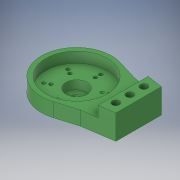
# Autodesk Inventor part: 000.403 - Рычаг
Saved by Autodesk Inventor 2019 (Build 230136000, 136)
## iProperties
Created: 2020-02-28
Part Number: 000.403 - Рычаг
Material: Пластик АБС
Document SubType Name: Modeling
Designer: Петров Иван
Density: 1.06 g/cm^3
Appearance: Гладкий — темный травянисто-зеленый
Author: Петров Иван
Autodesk Inventor part; units mm, degrees
ref_plane "YZ Plane" through (0, 0, 0) normal (1, 0, 0) x (0, 1, 0)
ref_plane "XZ Plane" through (0, 0, 0) normal (0, 1, 0) x (-1, 0, 0)
ref_plane "XY Plane" through (0, 0, 0) normal (0, 0, 1) x (1, 0, 0)
sketch "Эскиз1" plane through (0, 0, 0) normal (0, 1, 0) x (-1, 0, 0)
  arc A0 (13.2517, 5.1196) -> (11.6396, 8.8847) centre (11.8859, 6.7625) ccw
  line L0 (11.6396, 8.8847) -> (3.5765, 5.9707)
  line L1 (3.5765, 5.9707) -> (2.1921, 14.0362)
  arc A1 (2.1921, 14.0362) -> (-1.8746, 14.5225) centre (0.0865, 13.6747) ccw
  line L2 (-1.8746, 14.5225) -> (-3.3825, 6.0827)
  line L3 (-3.3825, 6.0827) -> (-11.0596, 8.9165)
  arc A2 (-11.0596, 8.9165) -> (-13.5142, 5.6378) centre (-11.7994, 6.9122) ccw
  line L4 (-13.5142, 5.6378) -> (-6.959, 0.112)
  line L5 (-6.959, 0.112) -> (-13.2517, -5.1196)
  arc A3 (-13.2517, -5.1196) -> (-11.6396, -8.8847) centre (-11.8859, -6.7625) ccw
  line L6 (-11.6396, -8.8847) -> (-3.5765, -5.9707)
  line L7 (-3.5765, -5.9707) -> (-2.1921, -14.0362)
  arc A4 (-2.1921, -14.0362) -> (1.8746, -14.5225) centre (-0.0865, -13.6747) ccw
  line L8 (1.8746, -14.5225) -> (3.3825, -6.0827)
  line L9 (3.3825, -6.0827) -> (11.0596, -8.9165)
  arc A5 (11.0596, -8.9165) -> (13.5142, -5.6378) centre (11.7994, -6.9122) ccw
  line L10 (13.5142, -5.6378) -> (6.959, -0.112)
  line L11 (6.959, -0.112) -> (13.2517, 5.1196)
  circle A6 centre (6.6709, 3.7954) radius 1
  circle A7 centre (11.8859, 6.7625) radius 1
  circle A8 centre (9.2109, -5.3958) radius 1
  circle A9 centre (-0.0485, -7.6748) radius 1
  circle A10 centre (-0.0865, -13.6747) radius 1
  circle A11 centre (-9.2784, -5.2789) radius 1
  circle A12 centre (-6.6223, 3.8794) radius 1
  circle A13 centre (-11.7994, 6.9122) radius 1
  circle A14 centre (0.0675, 10.6748) radius 1
  circle A15 centre (0, 0) radius 4.75
  circle A16 centre (0.0865, 13.6747) radius 1
  circle A17 centre (0.0485, 7.6748) radius 1
  circle A18 centre (-9.2109, 5.3958) radius 1
  circle A19 centre (-11.8859, -6.7625) radius 1
  circle A20 centre (-6.6709, -3.7954) radius 1
  circle A21 centre (-0.0675, -10.6748) radius 1
  circle A22 centre (11.7994, -6.9122) radius 1
  circle A23 centre (6.6223, -3.8794) radius 1
  circle A24 centre (9.2784, 5.2789) radius 1
  circle A25 centre (0, 0) radius 1.875
  circle A26 centre (0, 0) radius 20
  circle A27 centre (0, 0) radius 17.5
  point P0 (0, 0)
  dimension "d0" = 40
  dimension "d1" = 35
  constraints: 28 centre point, 24 end point, 12 point on circle, 2 coincident
  measures "d0" diameter of A26
  measures "d1" diameter of A27
extrude "Выдавливание1" add sketch "Эскиз1" along normal blind 2 contours L11 L10 A5 L9 L8 A4 L7 L6 A3 L5 L4 A2 L3 L2 A1 L1 L0 A0 | A26 | A27
sketch "Эскиз2" plane through (0, 2, 0) normal (0, 1, 0) x (1, 0, 0)
  arc A0 (13.2517, 5.1196) -> (11.6396, 8.8847) centre (11.8859, 6.7625) ccw
  line L0 (11.6396, 8.8847) -> (3.5765, 5.9707)
  line L1 (3.5765, 5.9707) -> (2.1921, 14.0362)
  arc A1 (2.1921, 14.0362) -> (-1.8746, 14.5225) centre (0.0865, 13.6747) ccw
  line L2 (-1.8746, 14.5225) -> (-3.3825, 6.0827)
  line L3 (-3.3825, 6.0827) -> (-11.0596, 8.9165)
  arc A2 (-11.0596, 8.9165) -> (-13.5142, 5.6378) centre (-11.7994, 6.9122) ccw
  line L4 (-13.5142, 5.6378) -> (-6.959, 0.112)
  line L5 (-6.959, 0.112) -> (-13.2517, -5.1196)
  arc A3 (-13.2517, -5.1196) -> (-11.6396, -8.8847) centre (-11.8859, -6.7625) ccw
  line L6 (-11.6396, -8.8847) -> (-3.5765, -5.9707)
  line L7 (-3.5765, -5.9707) -> (-2.1921, -14.0362)
  arc A4 (-2.1921, -14.0362) -> (1.8746, -14.5225) centre (-0.0865, -13.6747) ccw
  line L8 (1.8746, -14.5225) -> (3.3825, -6.0827)
  line L9 (3.3825, -6.0827) -> (11.0596, -8.9165)
  arc A5 (11.0596, -8.9165) -> (13.5142, -5.6378) centre (11.7994, -6.9122) ccw
  line L10 (13.5142, -5.6378) -> (6.959, -0.112)
  line L11 (6.959, -0.112) -> (13.2517, 5.1196)
  circle A6 centre (6.6709, 3.7954) radius 1
  circle A7 centre (11.8859, 6.7625) radius 1
  circle A8 centre (9.2109, -5.3958) radius 1
  circle A9 centre (-0.0485, -7.6748) radius 1
  circle A10 centre (-0.0865, -13.6747) radius 1
  circle A11 centre (-9.2784, -5.2789) radius 1
  circle A12 centre (-6.6223, 3.8794) radius 1
  circle A13 centre (-11.7994, 6.9122) radius 1
  circle A14 centre (0.0675, 10.6748) radius 1
  circle A15 centre (0, 0) radius 4.75
  circle A16 centre (0.0865, 13.6747) radius 1
  circle A17 centre (0.0485, 7.6748) radius 1
  circle A18 centre (-9.2109, 5.3958) radius 1
  circle A19 centre (-11.8859, -6.7625) radius 1
  circle A20 centre (-6.6709, -3.7954) radius 1
  circle A21 centre (-0.0675, -10.6748) radius 1
  circle A22 centre (11.7994, -6.9122) radius 1
  circle A23 centre (6.6223, -3.8794) radius 1
  circle A24 centre (9.2784, 5.2789) radius 1
  circle A25 centre (0, 0) radius 1.875
  circle A26 centre (0, 0) radius 20
  circle A27 centre (0, 0) radius 17.5
  point P0 (0, 0)
  dimension "d4" = 40
  dimension "d5" = 35
  constraints: 28 centre point, 24 end point, 12 point on circle, 2 coincident
  measures "d4" diameter of A26
  measures "d5" diameter of A27
extrude "Выдавливание2" add sketch "Эскиз2" along normal blind 6 contours A26
sketch "Эскиз3" plane through (0, 0, 0) normal (0, -1, 0) x (1, 0, 0)
  circle A0 centre (0, 0) radius 20 projected
  line L0 (15.264, 12.9232) -> (15.264, -12.9232)
  line L1 (15.264, 12.9232) -> (35.264, 12.9232)
  line L2 (35.264, 12.9232) -> (35.264, -12.9232)
  line L3 (35.264, -12.9232) -> (15.264, -12.9232)
  line L4 (15.264, -12.9232) -> (15.264, 12.9232)
  dimension "d8" = 20
  constraints: 10 end point, 2 parallel, 2 point on circle, 1 horizontal, 1 perpendicular, 1 vertical
  measures "d8" distance of L2.end L3.end
extrude "Выдавливание3" add sketch "Эскиз3" against normal up to surface (8 mm away) contours A0 L1 L2 L3
sketch "Эскиз4" plane through (0, 0, 0) normal (0, -1, 0) x (1, 0, 0)
  line L0 (35.264, 0) -> (30.264, 0)
  circle A0 centre (30.264, 0) radius 2
  point P0 (0, 0)
  dimension "d17" = 5
  dimension "d18" = 4
  constraints: 2 end point, 1 centre point, 1 coincident, 1 horizontal
  measures "d17" distance of L0.start L0.end
  measures "d18" diameter of A0
extrude "Выдавливание4" cut sketch "Эскиз4" against normal through all
pattern_linear "Прямоуг.массив2" count 3 spacing 8 along (0, 0, 1) of "Выдавливание4" first direction both ways yes
chamfer "Фаска3" distance 11 angle 45 2 edges at (15.264, 4, -12.9232) (15.264, 4, 12.9232)
chamfer "Фаска4" distance 9 angle 45 2 edges at (26.264, 4, 12.9232) (26.264, 4, -12.9232)
sketch "Эскиз8" plane through (0, 8, 0) normal (0, 1, 0) x (1, 0, 0)
  line L0 (17.6524, 15.5384) -> (35.264, 12.9232) projected
  line L1 (35.264, 12.9232) -> (35.264, -12.9232) projected
  line L2 (35.264, -12.9232) -> (17.6524, -15.5384) projected
  line L3 (35.264, 12.9232) -> (17.6524, 15.5384) projected
  line L4 (26.4582, 14.2308) -> (26.4582, -14.2308)
  line L5 (17.6524, -15.5384) -> (35.264, -12.9232) projected
  circle A0 centre (30.264, 8) radius 2 projected
  circle A1 centre (30.264, 0) radius 2 projected
  circle A2 centre (30.264, -8) radius 2 projected
  point P0 (0, 0)
  constraints: 2 end point, 2 midpoint
extrude "Выдавливание8" add sketch "Эскиз8" along normal blind 6
sketch "Эскиз9" plane through (0, 2, 0) normal (0, 1, 0) x (1, 0, 0)
  circle A0 centre (0, 0) radius 9
  dimension "d44" = 18
  constraints: 1 centre point, 1 coincident
  measures "d44" diameter of A0
extrude "Выдавливание9" add sketch "Эскиз9" against normal blind 6
sketch "Эскиз10" plane through (0, 2, 0) normal (0, 1, 0) x (1, 0, 0)
  circle A0 centre (0, 0) radius 3
  dimension "d48" = 6
  constraints: 1 centre point, 1 coincident
  measures "d48" diameter of A0
extrude "Выдавливание10" cut sketch "Эскиз10" against normal through all
sketch "Эскиз11" plane through (0, 2, 0) normal (0, 1, 0) x (1, 0, 0)
  circle A0 centre (0, 0) radius 6
  dimension "d52" = 12
  constraints: 1 centre point, 1 coincident
  measures "d52" diameter of A0
extrude "Выдавливание11" cut sketch "Эскиз11" against normal blind 5
sketch "Эскиз12" plane through (0, 8, 0) normal (0, 1, 0) x (1, 0, 0)
  line L0 (26.4582, 14.2308) -> (26.4582, -14.2308) projected
  line L1 (26.4582, 0) -> (23.4582, 0)
  circle A0 centre (23.4582, 0) radius 2.5
  point P0 (0, 0)
  dimension "d56" = 3
  dimension "d57" = 5
  constraints: 2 end point, 1 centre point, 1 coincident, 1 horizontal, 1 midpoint
  measures "d56" distance of L1.start L1.end
  measures "d57" diameter of A0
extrude "Выдавливание12" cut sketch "Эскиз12" against normal through all
